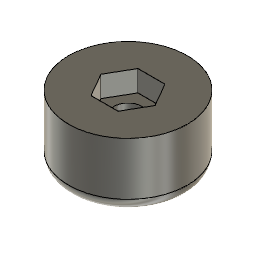
8) PLA Extrusion Feet (Autodesk Fusion 360 design; units mm, degrees)
Autodesk Fusion 360 part; units mm, degrees
ref_plane "WorkPlane1" through (0, 0, 0) normal (0, 0, 1) x (1, 0, 0)
sketch "Sketch1" plane through (0, 0, 0) normal (0, 0, 1) x (1, 0, 0)
  circle A0 centre (0, 0) radius 9
  dimension "d2" = 18
  constraint coincident A0.centre origin
  measures "d2" diameter of A0
extrude "Extrude1" add sketch "Sketch1" along normal blind 10
sketch "Sketch2" plane through (0, 0, 10) normal (0, 0, 1) x (-1, 0, 0)
  circle A0 centre (0, 0) radius 9
  line L0 (-2.0496, -3.55) -> (2.0496, -3.55)
  line L1 (2.0496, -3.55) -> (4.0992, 0)
  line L2 (4.0992, 0) -> (2.0496, 3.55)
  line L3 (2.0496, 3.55) -> (-2.0496, 3.55)
  line L4 (-2.0496, 3.55) -> (-4.0992, 0)
  line L5 (-4.0992, 0) -> (-2.0496, -3.55)
  dimension "d5" = 3.55
  constraint coincident A0.centre origin
  constraint horizontal L0
  measures "d5" distance of A0.centre L5
extrude "Extrude2" cut sketch "Sketch2" against normal blind 3.2 contours L0 L1 L2 L3 L4 L5
sketch "Sketch3" plane through (0, 0, 0) normal (0, 0, -1) x (1, 0, 0)
  circle A0 centre (0, 0) radius 9
  circle A1 centre (0, 0) radius 3.5
  dimension "d8" = 7
  constraint coincident A0.centre A1.centre
  measures "d8" diameter of A1
extrude "Extrude3" cut sketch "Sketch3" against normal blind 4.2 contours A1
sketch "Sketch4" plane through (0, 0, 4.2) normal (0, 0, -1) x (1, 0, 0)
  circle A0 centre (0, 0) radius 3.5
  circle A1 centre (0, 0) radius 2.1
  dimension "d11" = 4.2
  constraint concentric A0 A1
  measures "d11" diameter of A1
extrude "Extrude4" cut sketch "Sketch4" against normal up to surface (2.6 mm away) contours A1
fillet "Fillet1" radius 2 1 edges at (-8.3909, -3.2545, 0)
equation "d5 = ( 7.1 / 2 ) * 1 mm"
named bodies: "Extrusion M4 Bolt Shaker Base Feet"
